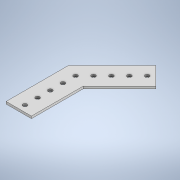
# Autodesk Inventor part: 135 Gusset
Saved by Autodesk Inventor 2021 (Build 250183000, 183)
## iProperties
Created: 2021-01-23
Part Number: 135 Gusset
Material: Generic
Document SubType Name: Modeling
Designer: aidan
Density: 1 g/cm^3
Appearance: Default
Author: aidan
Autodesk Inventor part; units mm, degrees
ref_plane "YZ Plane" through (0, 0, 0) normal (1, 0, 0) x (0, 1, 0)
ref_plane "XZ Plane" through (0, 0, 0) normal (0, 1, 0) x (-1, 0, 0)
ref_plane "XY Plane" through (0, 0, 0) normal (0, 0, 1) x (1, 0, 0)
sketch "Sketch1" plane through (0, 0, 0) normal (0, 1, 0) x (-1, 0, 0)
  line L0 (0, 0) -> (0, -62.2808)
  line L1 (0, -62.2808) -> (-44.0392, -106.32)
  line L2 (-44.0392, -106.32) -> (-61.9997, -88.3595)
  line L3 (-61.9997, -88.3595) -> (-25.4, -51.7598)
  line L4 (-25.4, -51.7598) -> (-25.4, 0)
  line L5 (-25.4, 0) -> (0, 0)
  line L6 (0, -62.2808) -> (-25.4, -51.7598) construction
  dimension "d0" = 62.2808
  dimension "d1" = 25.4
  dimension "d2" = 135
  constraints: 14 end point, 2 equal length, 2 parallel, 2 perpendicular, 1 vertical
  measures "d0" distance of L0.start L0.end
  measures "d1" distance of L4.end L0.start
  measures "d2" angle of L3 L4
extrude "Extrusion1" add sketch "Sketch1" along normal blind 2.286
sketch "Sketch2" plane through (0, 2.286, 0) normal (0, 1, 0) x (1, 0, 0)
  line L0 (44.0392, 106.32) -> (0, 62.2808) projected
  line L1 (25.4, 0) -> (25.4, 51.7598) projected
  line L2 (0, 62.2808) -> (25.4, 51.7598) construction
  point P0 (0, 0)
  point P1 (12.7, 57.0203)
  dimension "d5" = 12.7
  constraints: 2 end point, 1 midpoint
  measures "d5" distance from line of L1 point (12.7, 57.02)
hole "Hole1" at (12.7, 2.286, -57.0203) direction (0, -1, 0) diameter 4.1402 end through all
pattern_linear "Rectangular Pattern1" count 5 spacing 12.7 along (0, 0, 1) of "Hole1"
pattern_linear "Rectangular Pattern2" count 5 spacing 12.7 along (0.7071, 0, -0.7071) of "Hole1"
body "Solid1"
